Autodesk Inventor part; units mm, degrees
(part 2 of 2)
sketch "Skizze29" plane through (89.6, -2.4765, -33.8) normal (0, 0, -1) x (-1, 0, 0)
  line L0 (43.6, -0.4235) -> (43.6, -0.5235) construction
  line L1 (43.6, -0.5235) -> (49.9, -0.5235) construction
  line L2 (49.9, -0.5235) -> (52.9, 2.4765) construction
  line L3 (52.9, 2.4765) -> (79.4, 2.4765) construction
  line L4 (79.4, 2.4765) -> (79.4, 2.2765) construction
  line L5 (79.4, 2.2765) -> (83.4, 2.2765) construction
  line L6 (83.4, 2.2765) -> (83.4, 7.3765) construction
  line L7 (83.4, 7.3765) -> (49.9, 7.3765) construction
  line L8 (49.9, 7.3765) -> (49.9, 6.7966) construction
  line L9 (49.9, 6.7966) -> (45.4981, 2.3946) construction
  line L10 (45.4981, 2.3946) -> (38.1019, 2.3946) construction
  line L11 (38.1019, 2.3946) -> (33.7, 6.7966) construction
  line L12 (33.7, 6.7966) -> (33.7, 7.3765) construction
  line L13 (33.7, 7.3765) -> (17.2925, 7.3765) construction
  line L14 (17.2925, 7.3765) -> (17.2925, 2.4765) construction
  line L15 (17.2925, 2.4765) -> (31.9, 2.4765) construction
  line L16 (31.9, 2.4765) -> (34.8, -0.4235) construction
  line L17 (34.8, -0.4235) -> (43.6, -0.4235) construction
  line L18 (43.6, -28.4235) -> (34.8, -28.4235) construction
  line L19 (31.9, -31.3235) -> (34.8, -28.4235) construction
  line L20 (17.2925, -31.3235) -> (31.9, -31.3235) construction
  line L21 (17.2925, -31.3235) -> (17.2925, -36.2235) construction
  line L22 (33.7, -36.2235) -> (17.2925, -36.2235) construction
  line L23 (33.7, -36.2235) -> (33.7, -35.6437) construction
  line L24 (38.1019, -31.2417) -> (33.7, -35.6437) construction
  line L25 (45.4981, -31.2417) -> (38.1019, -31.2417) construction
  line L26 (49.9, -35.6437) -> (45.4981, -31.2417) construction
  line L27 (49.9, -35.6437) -> (49.9, -36.2235) construction
  line L28 (83.4, -36.2235) -> (49.9, -36.2235) construction
  line L29 (83.4, -31.1235) -> (83.4, -36.2235) construction
  line L30 (83.4, -31.1235) -> (79.4, -31.1235) construction
  line L31 (79.4, -31.3235) -> (79.4, -31.1235) construction
  line L32 (52.9, -31.3235) -> (79.4, -31.3235) construction
  line L33 (49.9, -28.3235) -> (52.9, -31.3235) construction
  line L34 (43.6, -28.3235) -> (49.9, -28.3235) construction
  line L35 (43.6, -28.3235) -> (43.6, -28.4235) construction
  line L36 (6, -28.8471) -> (0, -28.8471) construction
  line L37 (0, -28.8471) -> (0, -36.2235) construction
  line L38 (0, -36.2235) -> (6, -36.2235) construction
  line L39 (6, -36.2235) -> (6, -28.8471) construction
  line L40 (0, 7.3765) -> (0, 0) construction
  line L41 (0, 0) -> (6, 0) construction
  line L42 (6, 0) -> (6, 7.3765) construction
  line L43 (6, 7.3765) -> (0, 7.3765) construction
  line L44 (0, -28.8471) -> (3.8, -28.8471) construction
  line L45 (3.8, -27.1235) -> (3.8, -28.8471) construction
  line L46 (-4.5838, -27.1235) -> (3.8, -27.1235) construction
  line L47 (-4.5838, -1.7235) -> (-4.5838, -27.1235) construction
  line L48 (-4.5838, -1.7235) -> (3.8, -1.7235) construction
  line L49 (3.8, -1.7235) -> (3.8, 0) construction
  line L50 (3.8, 0) -> (0, 0) construction
  line L51 (0, 0) -> (0, 2.2765) construction
  line L52 (0, 2.2765) -> (-8.2, 2.2765) construction
  line L53 (-8.2, 2.2765) -> (-8.2, -31.1235) construction
  line L54 (0, -31.1235) -> (-8.2, -31.1235) construction
  line L55 (0, -31.1235) -> (0, -28.8471) construction
  line L56 (17.2925, 7.3765) -> (-8.2, 7.3765)
  line L57 (-8.2, 7.3765) -> (-8.2, -36.2235)
  line L58 (-8.2, -36.2235) -> (17.2925, -36.2235)
  line L59 (17.2925, -36.2235) -> (17.2925, 7.3765)
  line L60 (0, -36.2235) -> (6, -36.2235) projected
  point P0 (89.6, 2.4765)
  point P1 (3.8, 2.4765)
  constraints: 8 end point, 2 collinear, 2 parallel, 1 horizontal, 1 perpendicular
extrude "Extrusion29" cut sketch "Skizze29" against normal through all
sketch "Skizze30" plane through (0, 0, 0) normal (0, 0, 1) x (1, 0, 0)
  line L0 (72.3075, -38.7) -> (72.3075, -33.8) construction
  line L1 (57.7, -33.8) -> (72.3075, -33.8) construction
  line L2 (57.7, -33.8) -> (54.8, -30.9) construction
  line L3 (54.8, -30.9) -> (42, -30.9) construction
  line L4 (42, -30.9) -> (42, -30.8) construction
  line L5 (42, -30.8) -> (39.7, -30.8) construction
  line L6 (39.7, -30.8) -> (36.7, -33.8) construction
  line L7 (10.2, -33.8) -> (36.7, -33.8) construction
  line L8 (10.2, -29.4029) -> (10.2, -33.8) construction
  arc A0 (10.2, -4.3971) -> (10.2, -29.4029) centre (14.0958, -16.9) ccw construction
  line L9 (10.2, -4.3971) -> (10.2, 0) construction
  line L10 (10.2, 0) -> (36.7, 0) construction
  line L11 (39.7, -3) -> (36.7, 0) construction
  line L12 (42, -3) -> (39.7, -3) construction
  line L13 (42, -3) -> (42, -2.9) construction
  line L14 (42, -2.9) -> (54.8, -2.9) construction
  line L15 (57.7, 0) -> (54.8, -2.9) construction
  line L16 (57.7, 0) -> (72.3075, 0) construction
  line L17 (72.3075, 0) -> (72.3075, 4.9) construction
  line L18 (72.3075, 4.9) -> (55.9, 4.9) construction
  line L19 (55.9, 4.9) -> (55.9, 4.3201) construction
  line L20 (51.4981, -0.0818) -> (55.9, 4.3201) construction
  line L21 (44.1019, -0.0818) -> (51.4981, -0.0818) construction
  line L22 (39.7, 4.3201) -> (44.1019, -0.0818) construction
  line L23 (39.7, 4.3201) -> (39.7, 4.9) construction
  line L24 (39.7, 4.9) -> (6.2, 4.9) construction
  line L25 (6.2, 4.9) -> (6.2, -0.2) construction
  line L26 (6.2, -0.2) -> (-2, -0.2) construction
  line L27 (-2, -0.2) -> (-2, -33.6) construction
  line L28 (6.2, -33.6) -> (-2, -33.6) construction
  line L29 (6.2, -38.7) -> (6.2, -33.6) construction
  line L30 (39.7, -38.7) -> (6.2, -38.7) construction
  line L31 (39.7, -38.7) -> (39.7, -38.1201) construction
  line L32 (39.7, -38.1201) -> (44.1019, -33.7182) construction
  line L33 (44.1019, -33.7182) -> (51.4981, -33.7182) construction
  line L34 (51.4981, -33.7182) -> (55.9, -38.1201) construction
  line L35 (55.9, -38.1201) -> (55.9, -38.7) construction
  line L36 (72.3075, -38.7) -> (55.9, -38.7) construction
  circle A1 centre (59.1, -36.25) radius 1.4
  line L37 (-16.8615, -16.9) -> (87.169, -16.9) construction
  circle A2 centre (59.1, 2.45) radius 1.4
  line L38 (72.3075, -38.7) -> (72.3075, -33.8) construction
  line L39 (72.3075, -36.25) -> (54.0299, -36.25) construction
  line L40 (51.4981, -33.7182) -> (55.9, -38.1201) construction
  line L41 (57.7, -33.8) -> (54.8, -30.9) construction
  line L42 (57.7, -33.8) -> (57.7, -38.7) construction
  point P0 (0, 0)
  dimension "d149" = 2.8
  constraints: 4 end point, 3 point on line, 2 centre point, 1 horizontal, 1 midpoint, 1 symmetric about line, 1 tangent, 1 vertical, 1 other
  measures "d149" diameter of A1
extrude "Extrusion30" cut sketch "Skizze30" against normal through all
fillet "Rundung1" radius 3 2 edges at (72.3075, -38.7, -3) (72.3075, 4.9, -3)
sketch "Skizze31" plane through (0, 0, 0) normal (0, 0, 1) x (1, 0, 0)
  circle A0 centre (59.1, -36.25) radius 1.4 construction
  circle A1 centre (59.1, 2.45) radius 1.4 construction
  arc A2 (72.3075, 1.9) -> (69.3075, 4.9) centre (69.3075, 1.9) ccw construction
  line L0 (69.3075, 4.9) -> (55.9, 4.9) construction
  line L1 (55.9, 4.9) -> (55.9, 4.3201) construction
  line L2 (51.4981, -0.0818) -> (55.9, 4.3201) construction
  line L3 (44.1019, -0.0818) -> (51.4981, -0.0818) construction
  line L4 (39.7, 4.3201) -> (44.1019, -0.0818) construction
  line L5 (39.7, 4.3201) -> (39.7, 4.9) construction
  line L6 (39.7, 4.9) -> (6.2, 4.9) construction
  line L7 (6.2, 4.9) -> (6.2, -0.2) construction
  line L8 (6.2, -0.2) -> (-2, -0.2) construction
  line L9 (-2, -0.2) -> (-2, -33.6) construction
  line L10 (6.2, -33.6) -> (-2, -33.6) construction
  line L11 (6.2, -38.7) -> (6.2, -33.6) construction
  line L12 (39.7, -38.7) -> (6.2, -38.7) construction
  line L13 (39.7, -38.7) -> (39.7, -38.1201) construction
  line L14 (39.7, -38.1201) -> (44.1019, -33.7182) construction
  line L15 (44.1019, -33.7182) -> (51.4981, -33.7182) construction
  line L16 (51.4981, -33.7182) -> (55.9, -38.1201) construction
  line L17 (55.9, -38.1201) -> (55.9, -38.7) construction
  line L18 (69.3075, -38.7) -> (55.9, -38.7) construction
  arc A3 (69.3075, -38.7) -> (72.3075, -35.7) centre (69.3075, -35.7) ccw construction
  line L19 (72.3075, -35.7) -> (72.3075, -33.8) construction
  line L20 (57.7, -33.8) -> (72.3075, -33.8) construction
  line L21 (57.7, -33.8) -> (54.8, -30.9) construction
  line L22 (54.8, -30.9) -> (42, -30.9) construction
  line L23 (42, -30.9) -> (42, -30.8) construction
  line L24 (42, -30.8) -> (39.7, -30.8) construction
  line L25 (39.7, -30.8) -> (36.7, -33.8) construction
  line L26 (10.2, -33.8) -> (36.7, -33.8) construction
  line L27 (10.2, -29.4029) -> (10.2, -33.8) construction
  arc A4 (10.2, -4.3971) -> (10.2, -29.4029) centre (14.0958, -16.9) ccw construction
  line L28 (10.2, -4.3971) -> (10.2, 0) construction
  line L29 (10.2, 0) -> (36.7, 0) construction
  line L30 (39.7, -3) -> (36.7, 0) construction
  line L31 (42, -3) -> (39.7, -3) construction
  line L32 (42, -3) -> (42, -2.9) construction
  line L33 (42, -2.9) -> (54.8, -2.9) construction
  line L34 (57.7, 0) -> (54.8, -2.9) construction
  line L35 (57.7, 0) -> (72.3075, 0) construction
  line L36 (72.3075, 0) -> (72.3075, 1.9) construction
  line L37 (6.2, 4.9) -> (39.8, 4.9)
  line L38 (39.8, 4.9) -> (39.8, 8)
  line L39 (39.8, 8) -> (6.2, 8)
  line L40 (6.2, 8) -> (6.2, 4.9)
  line L41 (-16.9858, -16.9) -> (87.9146, -16.9) projected
  line L42 (39.7, -38.1201) -> (39.7, -38.7) construction
  line L43 (39.7, -38.7) -> (6.2, -38.7) construction
  line L44 (6.2, -38.7) -> (39.8, -38.7)
  line L45 (39.8, -38.7) -> (39.8, -41.8)
  line L46 (39.8, -41.8) -> (6.2, -41.8)
  line L47 (6.2, -41.8) -> (6.2, -38.7)
  point P0 (0, 0)
  dimension "d153" = 33.6
  dimension "d154" = 49.8
  constraints: 20 end point, 3 symmetric about line, 2 parallel, 1 horizontal, 1 perpendicular
  measures "d153" distance of L38.end L39.end
  measures "d154" distance between parallel lines of L46 L39
extrude "Extrusion31" add sketch "Skizze31" against normal up to surface (6 mm away)
sketch "Sketch40" plane through (0, 0, 0) normal (0, 0, 1) x (1, 0, 0)
  arc A0 (72.3075, 1.9) -> (69.3075, 4.9) centre (69.3075, 1.9) ccw construction
  line L0 (69.3075, 4.9) -> (55.9, 4.9) construction
  line L1 (44.1019, -0.0818) -> (51.4981, -0.0818) construction
  line L2 (39.7, 4.3201) -> (44.1019, -0.0818) construction
  line L3 (39.7, 4.3201) -> (39.7, 4.9) construction
  line L4 (39.7, 4.9) -> (39.8, 4.9) construction
  line L5 (39.8, 4.9) -> (39.8, 8) construction
  line L6 (39.8, 8) -> (6.2, 8) construction
  line L7 (6.2, 8) -> (6.2, -0.2) construction
  line L8 (6.2, -0.2) -> (-2, -0.2) construction
  line L9 (-2, -0.2) -> (-2, -33.6) construction
  line L10 (6.2, -33.6) -> (-2, -33.6) construction
  line L11 (6.2, -41.8) -> (6.2, -33.6) construction
  line L12 (39.8, -41.8) -> (6.2, -41.8) construction
  line L13 (39.8, -38.7) -> (39.8, -41.8) construction
  line L14 (39.7, -38.7) -> (39.8, -38.7) construction
  line L15 (39.7, -38.7) -> (39.7, -38.1201) construction
  line L16 (39.7, -38.1201) -> (44.1019, -33.7182) construction
  line L17 (44.1019, -33.7182) -> (51.4981, -33.7182) construction
  line L18 (69.3075, -38.7) -> (55.9, -38.7) construction
  arc A1 (69.3075, -38.7) -> (72.3075, -35.7) centre (69.3075, -35.7) ccw construction
  line L19 (72.3075, -35.7) -> (72.3075, -33.8) construction
  line L20 (57.7, -33.8) -> (72.3075, -33.8) construction
  line L21 (57.7, -33.8) -> (54.8, -30.9) construction
  line L22 (54.8, -30.9) -> (42, -30.9) construction
  line L23 (42, -30.9) -> (42, -30.8) construction
  line L24 (42, -30.8) -> (39.7, -30.8) construction
  line L25 (39.7, -30.8) -> (36.7, -33.8) construction
  line L26 (10.2, -33.8) -> (36.7, -33.8) construction
  line L27 (10.2, -29.4029) -> (10.2, -33.8) construction
  arc A2 (10.2, -4.3971) -> (10.2, -29.4029) centre (14.0958, -16.9) ccw construction
  line L28 (10.2, -4.3971) -> (10.2, 0) construction
  line L29 (10.2, 0) -> (36.7, 0) construction
  line L30 (39.7, -3) -> (36.7, 0) construction
  line L31 (42, -3) -> (39.7, -3) construction
  line L32 (42, -3) -> (42, -2.9) construction
  line L33 (42, -2.9) -> (54.8, -2.9) construction
  line L34 (57.7, 0) -> (54.8, -2.9) construction
  line L35 (57.7, 0) -> (72.3075, 0) construction
  line L36 (72.3075, 0) -> (72.3075, 1.9) construction
  line L37 (-16.9858, -16.9) -> (87.9146, -16.9) construction
  line L38 (6.2, 8) -> (6.2, 4.2406) construction
  line L39 (6.2, 4.2406) -> (1.7594, -0.2) construction
  line L40 (42, -12.2664) -> (34.1307, -4.3971) construction
  line L41 (1.7594, -0.2) -> (-2, -0.2) construction
  line L42 (6.2, -0.2) -> (-2, -0.2) construction
  line L43 (6.2, 4.2406) -> (1.7594, -0.2)
  line L44 (6.2, 8) -> (6.2, -0.2) projected
  line L45 (1.7594, -0.2) -> (6.2, -0.2)
  line L46 (6.2, -0.2) -> (6.2, 4.2406)
  line L47 (6.2, -33.6) -> (-2, -33.6) construction
  line L48 (6.2, -38.0406) -> (1.7594, -33.6) construction
  line L49 (1.7594, -33.6) -> (-2, -33.6) construction
  line L50 (6.2, -33.6) -> (-2, -33.6) construction
  line L51 (6.2, -38.0406) -> (1.7594, -33.6)
  line L52 (1.7594, -33.6) -> (6.2, -33.6)
  line L53 (6.2, -33.6) -> (6.2, -38.0406)
  line L54 (55.9, 4.9) -> (55.9, 4.3201) projected
  line L55 (51.4981, -0.0818) -> (55.9, 4.3201) projected
  line L56 (51.4981, -33.7182) -> (55.9, -38.1201) projected
  line L57 (55.9, -38.1201) -> (55.9, -38.7) projected
  point P0 (0, 0)
  point P1 (0, -33.8)
  dimension "d179" = 6.28
  constraints: 26 end point, 5 symmetric about line, 3 perpendicular, 1 collinear, 1 horizontal, 1 point on line
  measures "d179" distance of L38.end L39.end
extrude "Extrusion39" add sketch "Sketch40" against normal up to surface (6 mm away)
ref_plane "Work Plane5" through (6, -38.3, -33.8) normal (0, 0, -1) x (1, 0, 0)
ref_plane "Work Plane6" through (10.2, -29.4, -20.3) normal (0, 0, 1) x (-1, 0, 0)
ref_plane "Work Plane7" through (0, -33.8, -18) normal (0, 0, 1) x (-1, 0, 0)
body "Solid1"
